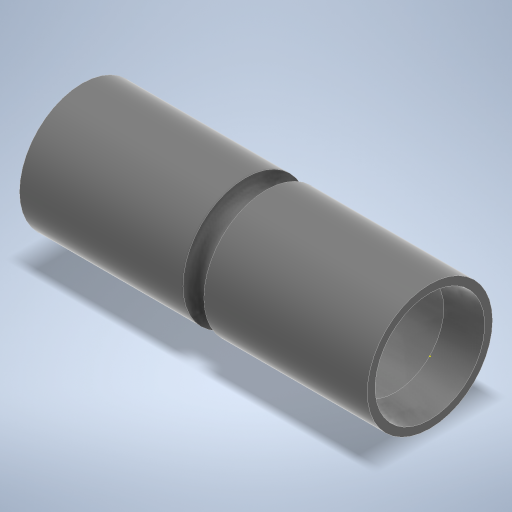
# Autodesk Inventor part: 01
Saved by Autodesk Inventor 2023 (Build 270158000, 158)
## iProperties
Created: 2023-09-01
Part Number: 01
Material: Genérico
Document SubType Name: Modeling
Designer: User
Density: 1 g/cm^3
Appearance: Suave - Preto
Author: User
Autodesk Inventor part; units mm, degrees
ref_plane "YZ Plane" through (0, 0, 0) normal (1, 0, 0) x (0, 1, 0)
ref_plane "XZ Plane" through (0, 0, 0) normal (0, 1, 0) x (-1, 0, 0)
ref_plane "XY Plane" through (0, 0, 0) normal (0, 0, 1) x (1, 0, 0)
sketch "Esboço1" plane through (0, 0, 0) normal (1, 0, 0) x (0, 1, 0)
  point P0 (0, 0)
sketch "Esboço2" plane through (0, 0, 0) normal (0, 0, 1) x (1, 0, 0)
  line L0 (0, 0) -> (-50, 0)
  arc A0 (-26.5, 9) -> (-23.5, 9) centre (-25, 9) ccw
  line L1 (0, 9) -> (-23.5, 9)
  line L2 (-26.5, 9) -> (-50, 9)
  line L3 (-45, 7) -> (-5, 7)
  line L4 (-50, 7.8816) -> (-50, 9)
  line L5 (-5, 7) -> (0, 7.8816)
  line L6 (-45, 7) -> (-50, 7.8816)
  line L7 (0, 9) -> (0, 7.8816)
  dimension "d4" = 50
  dimension "d6" = 3
  dimension "d11" = 10
  dimension "d14" = 5
  dimension "d17" = 10
  dimension "d19" = 5
  dimension "d20" = 14
  dimension "d21" = 18
  constraints: 16 end point, 2 point on circle, 1 centre point, 1 horizontal, 1 perpendicular, 1 vertical
  measures "d4" distance of L0.start L0.end
  measures "d6" diameter of A0
  measures "d11" angle of L5 L3
  measures "d14" horizontal distance of L5.end L3.end
  measures "d17" angle of L3 L6
  measures "d19" horizontal distance of L3.start L4.start
  measures "d20" diameter of L3 L0
  measures "d21" diameter of L2 L0
revolve "Revolução1" add sketch "Esboço2" angle 360 about axis through (0, 0, 0) along (-1, 0, 0)
